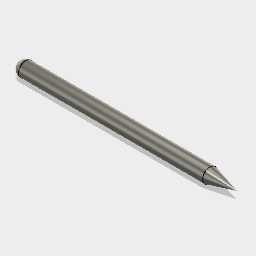
铅笔 (Autodesk Fusion 360 design; units mm, degrees)
Autodesk Fusion 360 part; units mm, degrees
cylinder "圆柱体基本要素1" add diameter 8 height 100 placed x (0, 0, -1) y (0, 1, 0) z (1, 0, 0) at (0, 13.8457, 17.0036) makes body 1
sphere "球体基本要素1" add diameter 8 placed x (0, 0, -1) y (0, 1, 0) z (1, 0, 0) at (0, 35, 30) separate body makes body 2
move_body "MoveFace1" bodies 2 to x (1, 0, 0) y (0, 1, 0) z (0, 0, 1) at (-9.0263, -19.6952, 0.948) on bodies 2
move_body "对齐1" bodies 2 to x (1, 0, 0) y (0, 1, 0) z (0, 0, 1) at (9.0263, -1.459, -17.9444)
move_body "对齐2" bodies 2 to x (1, 0, 0) y (0, 1, 0) z (0, 0, 1) at (0, 0, 4)
sketch "草图3" plane through (0, 0, 0) normal (1, 0, 0) x (0, 0, -1)
  line L0 (22.567, 13.8287) -> (18.567, 13.8287)
  line L1 (22.567, 13.8287) -> (22.567, -1.1713)
  line L2 (18.567, 13.8287) -> (22.567, -1.1713)
sketch "草图4" plane through (0, 0, 0) normal (0, 1, 0) x (1, 0, 0)
  line L0 (-53.5917, -11.509) -> (-53.0452, -15.4715)
  line L1 (-53.0452, -15.4715) -> (-38.1859, -13.422)
  line L2 (-53.5917, -11.509) -> (-38.1859, -13.422)
revolve "旋转2" add sketch "草图4" angle 360 about axis through (-53.0452, 0, 15.4715) along (0.990621, 0, -0.136637) separate body makes body 3
move_body "对齐3" bodies 3 to x (0.990621, 0, 0.136637) y (0, 1, 0) z (-0.136637, 0, 0.990621) at (154.6617, 0, 7.4306)
move_body "对齐4" bodies 3 to x (1, 0, 0) y (0, 1, 0) z (0, 0, 1) at (0, 13.8457, 1.4945)
combine "合并1" operation add target body 3 tool bodies 1 2
